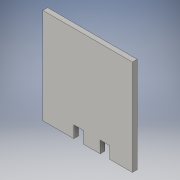
# Autodesk Inventor part: SideWall
Saved by Autodesk Inventor 2016 (Build 200138000, 138)
## iProperties
Created: 2016-05-26
Part Number: SideWall
Material: Generic
Document SubType Name: Modeling
Designer: cutrones
Density: 1 g/cm^3
Appearance: Default
Quanitity: 2
Width: 9.375 in
Author: cutrones
Autodesk Inventor part; units mm, degrees
ref_plane "YZ Plane" through (0, 0, 0) normal (1, 0, 0) x (0, 1, 0)
ref_plane "XZ Plane" through (0, 0, 0) normal (0, 1, 0) x (-1, 0, 0)
ref_plane "XY Plane" through (0, 0, 0) normal (0, 0, 1) x (1, 0, 0)
sketch "Sketch1" plane through (0, 0, 0) normal (0, 0, 1) x (1, 0, 0)
  point P0 (0, 0)
sketch "Sketch2" plane through (0, 0, 0) normal (0, 0, 1) x (1, 0, 0)
  line L0 (0, 0) -> (238.125, 0)
  line L1 (238.125, 0) -> (238.125, 254)
  line L2 (238.125, 254) -> (0, 254)
  line L3 (0, 254) -> (0, 0)
  line L4 (82.55, 0) -> (107.95, 0)
  line L5 (107.95, 0) -> (107.95, 31.75)
  line L6 (107.95, 31.75) -> (82.55, 31.75)
  line L7 (82.55, 31.75) -> (82.55, 0)
  line L8 (152.4, 0) -> (177.8, 0)
  line L9 (177.8, 0) -> (177.8, 31.75)
  line L10 (177.8, 31.75) -> (152.4, 31.75)
  line L11 (152.4, 31.75) -> (152.4, 0)
  line L12 (130.175, 254) -> (130.175, 0)
  dimension "Width" = 238.125
  dimension "d1" = 254
  dimension "d2" = 130.175
  dimension "d3" = 22.225
  dimension "d4" = 25.4
  dimension "d5" = 22.225
  dimension "d6" = 25.4
  dimension "d7" = 31.75
  constraints: 26 end point, 6 parallel, 5 point on line, 4 perpendicular, 3 horizontal
  measures "Width" distance of L2.end L1.end
  measures "d1" distance of L0.end L1.end
  measures "d2" distance between parallel lines of L12 L3
  measures "d3" distance between parallel lines of L12 L5
  measures "d4" distance between parallel lines of L7 L5
  measures "d5" distance between parallel lines of L11 L12
  measures "d6" distance between parallel lines of L9 L11
  measures "d7" distance between parallel lines of L8 L10
extrude "Extrusion1" add sketch "Sketch2" along normal blind 12.7 contours L3 L2 L12 L0 L5 L6 L7 | L2 L1 L0 L9 L10 L11 L12
equation "\"d1\" = Height"
equation "\"d8\" = Thick"
equation "\"Height\" = 254"
equation "\"Thick\" = 12.7"
body "Solid1"
